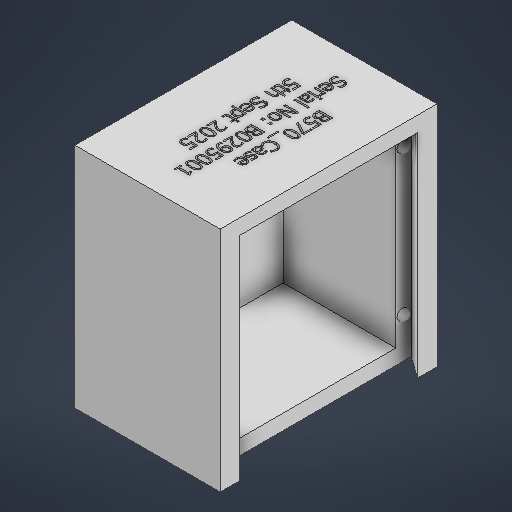
# Autodesk Inventor part: BoxCover295
Saved by Autodesk Inventor 2026.1 (Build 301233000, 233)
## iProperties
Created: 2025-09-05
Part Number: BoxCover295
Material: Generic
Document SubType Name: Modeling
Designer: usman
Density: 1 g/cm^3
Appearance: Default
Author: usman
Autodesk Inventor part; units mm, degrees
(part 1 of 2)
ref_plane "YZ Plane" through (0, 0, 0) normal (1, 0, 0) x (0, 1, 0)
ref_plane "XZ Plane" through (0, 0, 0) normal (0, 1, 0) x (-1, 0, 0)
ref_plane "XY Plane" through (0, 0, 0) normal (0, 0, 1) x (1, 0, 0)
sketch "Sketch1" plane through (0, 0, 0) normal (1, 0, 0) x (0, 1, 0)
  line L0 (-52.5, 50) -> (52.5, 50)
  line L1 (52.5, 50) -> (52.5, -50)
  line L2 (52.5, -50) -> (-52.5, -50)
  line L3 (-52.5, -50) -> (-52.5, 50)
  line L4 (-52.5, 50) -> (52.5, -50) construction
  line L5 (52.5, 50) -> (-52.5, -50) construction
  point P0 (0, 0)
  dimension "d0" = 100
  dimension "d1" = 105
  constraints: 12 end point, 2 midpoint, 2 parallel, 1 horizontal, 1 perpendicular
  measures "d0" distance of L0.end L1.end
  measures "d1" distance of L1.end L2.end
extrude "Extrusion1" add sketch "Sketch1" along normal blind 67
sketch "Sketch2" plane through (67, 0, 0) normal (1, 0, 0) x (0, 0, -1)
  line L0 (-41, -45.5) -> (41, -45.5)
  line L1 (41, -45.5) -> (41, 45.5)
  line L2 (41, 45.5) -> (-41, 45.5)
  line L3 (-41, 45.5) -> (-41, -45.5)
  line L4 (-41, -45.5) -> (41, 45.5) construction
  line L5 (41, -45.5) -> (-41, 45.5) construction
  point P0 (0, 0)
  dimension "d4" = 82
  dimension "d5" = 91
  constraints: 12 end point, 2 midpoint, 2 parallel, 1 horizontal, 1 perpendicular
  measures "d4" distance of L1.end L2.end
  measures "d5" distance of L0.end L1.end
extrude "Extrusion2" cut sketch "Sketch2" against normal blind 62
sketch "Sketch3" plane through (0, -52.5, -50) normal (0, -1, 0) x (1, 0, 0)
  point P0 (0, 50)
sketch "Sketch4" plane through (0, -52.5, -50) normal (0, -1, 0) x (1, 0, 0)
  point P0 (0, 50)
sketch "Sketch9" plane through (0, -52.5, -50) normal (0, -1, 0) x (1, 0, 0)
  line L0 (67, 9) -> (67, 91) projected
  line L1 (67, 91) -> (57, 98.0021)
  line L2 (57, 98.0021) -> (57, 1.9979)
  line L3 (57, 1.9979) -> (67, 9)
  line L4 (67, 100) -> (67, 0) projected
  point P0 (0, 50)
  dimension "d14" = 125
  dimension "d15" = 10
  dimension "d16" = 125
  constraints: 6 end point, 1 parallel
  measures "d14" angle of L4 L1
  measures "d15" distance from line of L2 L0.end
  measures "d16" angle of L3 L4
extrude "Extrusion3" cut sketch "Sketch9" against normal up to surface (98 mm away)
sketch "Sketch10" plane through (57, -52.5, 48.0021) normal (1, 0, 0) x (0, 0, -1)
  arc A0 (6.5021, 86) -> (1.5021, 86) centre (4.0021, 86) ccw
  arc A1 (94.5021, 86) -> (89.5021, 86) centre (92.0021, 86) ccw
  line L0 (7.0021, 98) -> (0, 98) projected
  line L1 (96.0042, 98) -> (89.0021, 98) projected
  line L2 (89.0021, 98) -> (89.0021, 0) projected
  line L3 (7.0021, 0) -> (7.0021, 98) projected
  line L4 (1.5021, 86) -> (6.5021, 86)
  line L5 (0, 0) -> (0, 98) projected
  line L6 (89.5021, 86) -> (94.5021, 86)
  point P0 (48.0021, 52.5)
  point P1 (3.501, 98)
  point P2 (92.5031, 98)
  dimension "d19" = 5
  dimension "d20" = 5
  dimension "d21" = 12
  dimension "d22" = 12
  dimension "d23" = 3
  dimension "d24" = 3
  constraints: 4 end point, 4 point on circle, 2 centre point, 2 midpoint, 1 horizontal, 1 perpendicular, 1 other
  measures "d19" diameter of A0
  measures "d20" diameter of A1
  measures "d21" vertical distance of point (3.501, 98) A0.centre
  measures "d22" vertical distance of point (92.503, 98) A1.centre
  measures "d23" distance from line of L2 A1.centre
  measures "d24" distance from line of L3 A0.centre
revolve "Revolution1" add sketch "Sketch10" angle 360 about axis through (57, 33.5, -41.5) along (0, 0, -1)
sketch "Sketch11" plane through (0, 52.5, 50) normal (0, 1, 0) x (1, 0, 0)
  line L0 (68.0097, 100.1192) -> (68.0097, 0.8322) construction
  line L1 (68.0097, 0.8322) -> (1.2743, 0.8322) construction
  line L2 (1.2743, 0.8322) -> (1.2743, 100.1192) construction
  line L3 (1.2743, 100.1192) -> (68.0097, 100.1192) construction
  spline S0 degree 2 poles (44.2837, 66.1356) (43.8292, 66.1356) (43.1327, 66.4814) (42.9055, 66.768) knots 0 0 0 1 2 2 2
  spline S1 degree 2 poles (42.9055, 66.768) (42.6387, 67.1138) (42.4115, 67.8992) (42.4115, 68.5217) knots 0 0 0 1 2 2 2
  line L4 (42.4115, 68.5217) -> (42.4115, 70.2704)
  line L5 (42.4115, 70.2704) -> (48.5075, 70.2704)
  line L6 (48.5075, 70.2704) -> (48.5075, 68.655)
  spline S2 degree 2 poles (48.5075, 68.655) (48.5075, 68.003) (48.4235, 67.3509) (48.2605, 67.0545) knots 0 0 0 1 2 2 2
  spline S3 degree 2 poles (48.2605, 67.0545) (48.0875, 66.7235) (47.5194, 66.4222) (47.1341, 66.4222) knots 0 0 0 1 2 2 2
  spline S4 degree 2 poles (47.1341, 66.4222) (46.7043, 66.4222) (46.0226, 66.8766) (45.83, 67.2768) knots 0 0 0 1 2 2 2
  line L7 (45.83, 67.2768) -> (45.8003, 67.2768)
  spline S5 degree 2 poles (45.8003, 67.2768) (45.6521, 66.7334) (44.8666, 66.1356) (44.2837, 66.1356) knots 0 0 0 1 2 2 2
  spline S6 degree 2 poles (44.2491, 66.9804) (44.5949, 66.9804) (45.0395, 67.178) (45.1976, 67.4744) knots 0 0 0 1 2 2 2
  spline S7 degree 2 poles (45.1976, 67.4744) (45.2964, 67.667) (45.3557, 68.1215) (45.3557, 68.5414) knots 0 0 0 1 2 2 2
  line L8 (45.3557, 68.5414) -> (45.3557, 69.4603)
  line L9 (45.3557, 69.4603) -> (43.1031, 69.4603)
  line L10 (43.1031, 69.4603) -> (43.1031, 68.8032)
  spline S8 degree 2 poles (43.1031, 68.8032) (43.1031, 68.2697) (43.2019, 67.6572) (43.3599, 67.42) knots 0 0 0 1 2 2 2
  spline S9 degree 2 poles (43.3599, 67.42) (43.523, 67.1928) (43.928, 66.9804) (44.2491, 66.9804) knots 0 0 0 1 2 2 2
  spline S10 degree 2 poles (47.0205, 67.2669) (47.2379, 67.2669) (47.5639, 67.4151) (47.6578, 67.5781) knots 0 0 0 1 2 2 2
  spline S11 degree 2 poles (47.6578, 67.5781) (47.7664, 67.7757) (47.8158, 68.2549) (47.8158, 68.6847) knots 0 0 0 1 2 2 2
  line L11 (47.8158, 68.6847) -> (47.8158, 69.4603)
  line L12 (47.8158, 69.4603) -> (46.0325, 69.4603)
  line L13 (46.0325, 69.4603) -> (46.0325, 68.5414)
  spline S12 degree 2 poles (46.0325, 68.5414) (46.0325, 68.161) (46.1115, 67.8004) (46.235, 67.6078) knots 0 0 0 1 2 2 2
  spline S13 degree 2 poles (46.235, 67.6078) (46.3536, 67.42) (46.734, 67.2669) (47.0205, 67.2669) knots 0 0 0 1 2 2 2
  spline S14 degree 2 poles (44.3479, 61.8082) (43.9083, 61.8082) (43.1574, 62.0897) (42.8808, 62.3466) knots 0 0 0 1 2 2 2
  spline S15 degree 2 poles (42.8808, 62.3466) (42.6041, 62.6035) (42.283, 63.3692) (42.283, 63.8435) knots 0 0 0 1 2 2 2
  spline S16 degree 2 poles (42.283, 63.8435) (42.283, 64.2782) (42.4757, 65.1279) (42.6288, 65.4391) knots 0 0 0 1 2 2 2
  line L14 (42.6288, 65.4391) -> (43.4933, 65.4391)
  line L15 (43.4933, 65.4391) -> (43.4933, 65.3798)
  spline S17 degree 2 poles (43.4933, 65.3798) (43.4242, 65.2859) (43.2463, 64.9352) (43.1673, 64.7228) knots 0 0 0 1 2 2 2
  spline S18 degree 2 poles (43.1673, 64.7228) (43.0833, 64.4807) (42.9894, 64.0806) (42.9894, 63.8286) knots 0 0 0 1 2 2 2
  spline S19 degree 2 poles (42.9894, 63.8286) (42.9894, 63.5816) (43.1673, 63.1173) (43.3599, 62.9493) knots 0 0 0 1 2 2 2
  spline S20 degree 2 poles (43.3599, 62.9493) (43.5427, 62.7962) (44.0268, 62.6381) (44.3529, 62.6381) knots 0 0 0 1 2 2 2
  spline S21 degree 2 poles (44.3529, 62.6381) (44.6789, 62.6381) (45.0939, 62.8159) (45.2322, 62.9839) knots 0 0 0 1 2 2 2
  spline S22 degree 2 poles (45.2322, 62.9839) (45.3854, 63.1568) (45.5138, 63.6706) (45.5138, 63.9818) knots 0 0 0 1 2 2 2
  spline S23 degree 2 poles (45.5138, 63.9818) (45.5138, 64.3177) (45.4101, 64.9846) (45.3656, 65.1871) knots 0 0 0 1 2 2 2
  line L16 (45.3656, 65.1871) -> (48.5075, 65.1871)
  line L17 (48.5075, 65.1871) -> (48.5075, 61.8427)
  line L18 (48.5075, 61.8427) -> (47.7911, 61.8427)
  line L19 (47.7911, 61.8427) -> (47.7911, 64.4017)
  line L20 (47.7911, 64.4017) -> (46.1659, 64.4017)
  spline S24 degree 2 poles (46.1659, 64.4017) (46.1856, 64.2535) (46.2005, 63.967) (46.2005, 63.8484) knots 0 0 0 1 2 2 2
  spline S25 degree 2 poles (46.2005, 63.8484) (46.2005, 63.3791) (46.0473, 62.732) (45.8201, 62.4355) knots 0 0 0 1 2 2 2
  spline S26 degree 2 poles (45.8201, 62.4355) (45.5928, 62.1342) (44.9012, 61.8082) (44.3479, 61.8082) knots 0 0 0 1 2 2 2
  line L21 (47.5935, 57.1003) -> (42.4115, 59.7383)
  line L22 (42.4115, 59.7383) -> (42.4115, 60.6077)
  line L23 (42.4115, 60.6077) -> (47.7911, 57.8216)
  line L24 (47.7911, 57.8216) -> (47.7911, 60.9684)
  line L25 (47.7911, 60.9684) -> (48.5075, 60.9684)
  line L26 (48.5075, 60.9684) -> (48.5075, 57.1003)
  line L27 (48.5075, 57.1003) -> (47.5935, 57.1003)
  spline S27 degree 2 poles (45.4595, 52.5604) (43.8194, 52.5604) (42.283, 53.5138) (42.283, 54.5068) knots 0 0 0 1 2 2 2
  spline S28 degree 2 poles (42.283, 54.5068) (42.283, 55.5146) (43.849, 56.4581) (45.4545, 56.4581) knots 0 0 0 1 2 2 2
  spline S29 degree 2 poles (45.4545, 56.4581) (47.1045, 56.4581) (48.631, 55.5047) (48.631, 54.5068) knots 0 0 0 1 2 2 2
  spline S30 degree 2 poles (48.631, 54.5068) (48.631, 53.504) (47.0501, 52.5604) (45.4595, 52.5604) knots 0 0 0 1 2 2 2
  spline S31 degree 2 poles (43.602, 53.6077) (43.9033, 53.4891) (44.8321, 53.3903) (45.4595, 53.3903) knots 0 0 0 1 2 2 2
  spline S32 degree 2 poles (45.4595, 53.3903) (46.0868, 53.3903) (47.0106, 53.4891) (47.3218, 53.6127) knots 0 0 0 1 2 2 2
  spline S33 degree 2 poles (47.3218, 53.6127) (47.6331, 53.7362) (47.9542, 54.1659) (47.9542, 54.5068) knots 0 0 0 1 2 2 2
  spline S34 degree 2 poles (47.9542, 54.5068) (47.9542, 54.8477) (47.6331, 55.2873) (47.312, 55.4158) knots 0 0 0 1 2 2 2
  spline S35 degree 2 poles (47.312, 55.4158) (47.0007, 55.5393) (46.0523, 55.6282) (45.4545, 55.6282) knots 0 0 0 1 2 2 2
  spline S36 degree 2 poles (45.4545, 55.6282) (44.8123, 55.6282) (43.9527, 55.5491) (43.6168, 55.4207) knots 0 0 0 1 2 2 2
  spline S37 degree 2 poles (43.6168, 55.4207) (43.3007, 55.3021) (42.9598, 54.8625) (42.9598, 54.5068) knots 0 0 0 1 2 2 2
  spline S38 degree 2 poles (42.9598, 54.5068) (42.9598, 54.1709) (43.2809, 53.7312) (43.602, 53.6077) knots 0 0 0 1 2 2 2
  line L28 (41.1863, 47.5858) -> (41.1863, 52.2887)
  line L29 (41.1863, 52.2887) -> (41.7149, 52.2887)
  line L30 (41.7149, 52.2887) -> (41.7149, 47.5858)
  line L31 (41.7149, 47.5858) -> (41.1863, 47.5858)
  spline S39 degree 2 poles (42.3028, 44.6514) (42.3028, 45.2442) (42.7029, 46.2471) (43.1031, 46.6126) knots 0 0 0 1 2 2 2
  spline S40 degree 2 poles (43.1031, 46.6126) (43.4983, 46.9782) (44.6839, 47.3783) (45.4545, 47.3783) knots 0 0 0 1 2 2 2
  spline S41 degree 2 poles (45.4545, 47.3783) (46.2202, 47.3783) (47.3564, 46.9881) (47.7763, 46.6176) knots 0 0 0 1 2 2 2
  spline S42 degree 2 poles (47.7763, 46.6176) (48.1864, 46.252) (48.6161, 45.2541) (48.6161, 44.6366) knots 0 0 0 1 2 2 2
  spline S43 degree 2 poles (48.6161, 44.6366) (48.6161, 44.3303) (48.5272, 43.7919) (48.4581, 43.5646) knots 0 0 0 1 2 2 2
  spline S44 degree 2 poles (48.4581, 43.5646) (48.3938, 43.367) (48.2111, 42.957) (48.1024, 42.7545) knots 0 0 0 1 2 2 2
  line L32 (48.1024, 42.7545) -> (47.1242, 42.7545)
  line L33 (47.1242, 42.7545) -> (47.1242, 42.8187)
  spline S45 degree 2 poles (47.1242, 42.8187) (47.223, 42.9274) (47.4997, 43.2633) (47.6331, 43.5053) knots 0 0 0 1 2 2 2
  spline S46 degree 2 poles (47.6331, 43.5053) (47.7615, 43.7375) (47.9245, 44.2859) (47.9245, 44.6416) knots 0 0 0 1 2 2 2
  spline S47 degree 2 poles (47.9245, 44.6416) (47.9245, 45.0318) (47.6034, 45.7284) (47.2971, 45.9902) knots 0 0 0 1 2 2 2
  spline S48 degree 2 poles (47.2971, 45.9902) (46.9859, 46.2471) (46.0424, 46.5336) (45.4545, 46.5336) knots 0 0 0 1 2 2 2
  spline S49 degree 2 poles (45.4545, 46.5336) (44.8271, 46.5336) (43.9231, 46.2322) (43.6119, 45.9704) knots 0 0 0 1 2 2 2
  spline S50 degree 2 poles (43.6119, 45.9704) (43.3105, 45.7135) (43.0043, 45.0269) (43.0043, 44.6416) knots 0 0 0 1 2 2 2
  spline S51 degree 2 poles (43.0043, 44.6416) (43.0043, 44.2908) (43.1772, 43.6931) (43.3056, 43.4609) knots 0 0 0 1 2 2 2
  spline S52 degree 2 poles (43.3056, 43.4609) (43.434, 43.2386) (43.7008, 42.9076) (43.7947, 42.8137) knots 0 0 0 1 2 2 2
  line L34 (43.7947, 42.8137) -> (43.7947, 42.7545)
  line L35 (43.7947, 42.7545) -> (42.8264, 42.7545)
  spline S53 degree 2 poles (42.8264, 42.7545) (42.7326, 42.957) (42.5597, 43.3127) (42.4806, 43.5646) knots 0 0 0 1 2 2 2
  spline S54 degree 2 poles (42.4806, 43.5646) (42.3917, 43.8314) (42.3028, 44.2859) (42.3028, 44.6514) knots 0 0 0 1 2 2 2
  spline S55 degree 2 poles (42.8956, 39.5089) (42.8264, 39.6027) (42.5794, 39.9189) (42.5053, 40.0671) knots 0 0 0 1 2 2 2
  spline S56 degree 2 poles (42.5053, 40.0671) (42.3966, 40.2696) (42.283, 40.65) (42.283, 40.9958) knots 0 0 0 1 2 2 2
  spline S57 degree 2 poles (42.283, 40.9958) (42.283, 41.2774) (42.4954, 41.7862) (42.6881, 41.9789) knots 0 0 0 1 2 2 2
  spline S58 degree 2 poles (42.6881, 41.9789) (42.8758, 42.1617) (43.4291, 42.384) (43.7354, 42.384) knots 0 0 0 1 2 2 2
  spline S59 degree 2 poles (43.7354, 42.384) (44.2096, 42.384) (44.8815, 41.9838) (45.0741, 41.5491) knots 0 0 0 1 2 2 2
  spline S60 degree 2 poles (45.0741, 41.5491) (45.252, 41.1638) (45.3854, 40.1165) (45.4199, 39.5089) knots 0 0 0 1 2 2 2
  line L36 (45.4199, 39.5089) -> (45.5681, 39.5089)
  spline S61 degree 2 poles (45.5681, 39.5089) (45.8349, 39.5089) (46.1659, 39.6719) (46.2597, 39.8201) knots 0 0 0 1 2 2 2
  spline S62 degree 2 poles (46.2597, 39.8201) (46.3536, 39.9683) (46.4129, 40.3931) (46.4129, 40.6204) knots 0 0 0 1 2 2 2
  spline S63 degree 2 poles (46.4129, 40.6204) (46.4129, 40.8871) (46.2548, 41.6084) (46.1017, 41.969) knots 0 0 0 1 2 2 2
  line L37 (46.1017, 41.969) -> (46.1017, 42.0135)
  line L38 (46.1017, 42.0135) -> (46.8871, 42.0135)
  spline S64 degree 2 poles (46.8871, 42.0135) (46.9464, 41.801) (47.0946, 41.0057) (47.0946, 40.6154) knots 0 0 0 1 2 2 2
  spline S65 degree 2 poles (47.0946, 40.6154) (47.0946, 40.1412) (46.9464, 39.494) (46.7537, 39.2372) knots 0 0 0 1 2 2 2
  spline S66 degree 2 poles (46.7537, 39.2372) (46.566, 38.9852) (45.9683, 38.7382) (45.5385, 38.7382) knots 0 0 0 1 2 2 2
  line L39 (45.5385, 38.7382) -> (42.4115, 38.7382)
  line L40 (42.4115, 38.7382) -> (42.4115, 39.5089)
  line L41 (42.4115, 39.5089) -> (42.8956, 39.5089)
  line L42 (43.5378, 39.5089) -> (44.8074, 39.5089)
  spline S67 degree 2 poles (44.8074, 39.5089) (44.7827, 39.7855) (44.6987, 40.6204) (44.6196, 40.8822) knots 0 0 0 1 2 2 2
  spline S68 degree 2 poles (44.6196, 40.8822) (44.5258, 41.1885) (44.1355, 41.5886) (43.7897, 41.5886) knots 0 0 0 1 2 2 2
  spline S69 degree 2 poles (43.7897, 41.5886) (43.3945, 41.5886) (42.9944, 41.144) (42.9944, 40.7192) knots 0 0 0 1 2 2 2
  spline S70 degree 2 poles (42.9944, 40.7192) (42.9944, 40.3585) (43.3056, 39.7657) (43.5378, 39.5089) knots 0 0 0 1 2 2 2
  spline S71 degree 2 poles (42.3028, 36.4213) (42.3028, 36.8808) (42.5498, 37.6761) (42.6881, 37.9379) knots 0 0 0 1 2 2 2
  line L43 (42.6881, 37.9379) -> (43.5526, 37.9379)
  line L44 (43.5526, 37.9379) -> (43.5526, 37.8984)
  spline S72 degree 2 poles (43.5526, 37.8984) (43.4736, 37.7996) (43.2858, 37.5328) (43.1821, 37.3105) knots 0 0 0 1 2 2 2
  spline S73 degree 2 poles (43.1821, 37.3105) (43.0882, 37.1179) (42.9499, 36.6436) (42.9499, 36.3917) knots 0 0 0 1 2 2 2
  spline S74 degree 2 poles (42.9499, 36.3917) (42.9499, 36.2089) (43.0339, 35.789) (43.1031, 35.6902) knots 0 0 0 1 2 2 2
  spline S75 degree 2 poles (43.1031, 35.6902) (43.1969, 35.547) (43.4093, 35.4185) (43.6267, 35.4185) knots 0 0 0 1 2 2 2
  spline S76 degree 2 poles (43.6267, 35.4185) (43.8984, 35.4185) (44.18, 35.7149) (44.2738, 36.0953) knots 0 0 0 1 2 2 2
  spline S77 degree 2 poles (44.2738, 36.0953) (44.3084, 36.2435) (44.4072, 36.7177) (44.4616, 36.9203) knots 0 0 0 1 2 2 2
  spline S78 degree 2 poles (44.4616, 36.9203) (44.6147, 37.4439) (45.247, 37.9182) (45.6966, 37.9182) knots 0 0 0 1 2 2 2
  spline S79 degree 2 poles (45.6966, 37.9182) (46.319, 37.9182) (47.0946, 36.9845) (47.0946, 36.2139) knots 0 0 0 1 2 2 2
  spline S80 degree 2 poles (47.0946, 36.2139) (47.0946, 35.8335) (46.9069, 35.0628) (46.7636, 34.801) knots 0 0 0 1 2 2 2
  line L45 (46.7636, 34.801) -> (45.9386, 34.801)
  line L46 (45.9386, 34.801) -> (45.9386, 34.8405)
  spline S81 degree 2 poles (45.9386, 34.8405) (46.1758, 35.1369) (46.4475, 35.8582) (46.4475, 36.2287) knots 0 0 0 1 2 2 2
  spline S82 degree 2 poles (46.4475, 36.2287) (46.4475, 36.6091) (46.1264, 37.1327) (45.8053, 37.1327) knots 0 0 0 1 2 2 2
  spline S83 degree 2 poles (45.8053, 37.1327) (45.5138, 37.1327) (45.2322, 36.8215) (45.1433, 36.4757) knots 0 0 0 1 2 2 2
  spline S84 degree 2 poles (45.1433, 36.4757) (45.0988, 36.3077) (45.0099, 35.8829) (44.9556, 35.6507) knots 0 0 0 1 2 2 2
  spline S85 degree 2 poles (44.9556, 35.6507) (44.8271, 35.1468) (44.2393, 34.633) (43.7304, 34.633) knots 0 0 0 1 2 2 2
  spline S86 degree 2 poles (43.7304, 34.633) (43.434, 34.633) (42.9104, 34.8652) (42.7177, 35.0925) knots 0 0 0 1 2 2 2
  spline S87 degree 2 poles (42.7177, 35.0925) (42.5152, 35.3345) (42.3028, 35.952) (42.3028, 36.4213) knots 0 0 0 1 2 2 2
  spline S88 degree 2 poles (42.3077, 31.9308) (42.3077, 33.0275) (43.5378, 34.2329) (44.674, 34.2329) knots 0 0 0 1 2 2 2
  spline S89 degree 2 poles (44.674, 34.2329) (45.7904, 34.2329) (47.1144, 33.0621) (47.1144, 32.1186) knots 0 0 0 1 2 2 2
  spline S90 degree 2 poles (47.1144, 32.1186) (47.1144, 31.6937) (46.8674, 31.0367) (46.6055, 30.7946) knots 0 0 0 1 2 2 2
  spline S91 degree 2 poles (46.6055, 30.7946) (46.3437, 30.5476) (45.5879, 30.2858) (45.0395, 30.2858) knots 0 0 0 1 2 2 2
  line L47 (45.0395, 30.2858) -> (44.6196, 30.2858)
  line L48 (44.6196, 30.2858) -> (44.6196, 33.4524)
  spline S92 degree 2 poles (44.6196, 33.4524) (43.8243, 33.4524) (42.9796, 32.6521) (42.9796, 31.9407) knots 0 0 0 1 2 2 2
  spline S93 degree 2 poles (42.9796, 31.9407) (42.9796, 31.6888) (43.0932, 31.1997) (43.1821, 31.0021) knots 0 0 0 1 2 2 2
  spline S94 degree 2 poles (43.1821, 31.0021) (43.2809, 30.7946) (43.4538, 30.5081) (43.5328, 30.4143) knots 0 0 0 1 2 2 2
  line L49 (43.5328, 30.4143) -> (43.5328, 30.3698)
  line L50 (43.5328, 30.3698) -> (42.693, 30.3698)
  spline S95 degree 2 poles (42.693, 30.3698) (42.6387, 30.5032) (42.4806, 30.9083) (42.4362, 31.0663) knots 0 0 0 1 2 2 2
  spline S96 degree 2 poles (42.4362, 31.0663) (42.3719, 31.2886) (42.3077, 31.6542) (42.3077, 31.9308) knots 0 0 0 1 2 2 2
  spline S97 degree 2 poles (45.2075, 31.0367) (45.5187, 31.0466) (45.9732, 31.175) (46.1264, 31.2985) knots 0 0 0 1 2 2 2
  spline S98 degree 2 poles (46.1264, 31.2985) (46.2993, 31.4319) (46.482, 31.8518) (46.482, 32.163) knots 0 0 0 1 2 2 2
  spline S99 degree 2 poles (46.482, 32.163) (46.482, 32.4693) (46.2993, 32.8991) (46.1214, 33.0769) knots 0 0 0 1 2 2 2
  spline S100 degree 2 poles (46.1214, 33.0769) (45.9386, 33.2498) (45.499, 33.4277) (45.2075, 33.4524) knots 0 0 0 1 2 2 2
  line L51 (45.2075, 33.4524) -> (45.2075, 31.0367)
  spline S101 degree 2 poles (32.2659, 85.9822) (32.2659, 86.6442) (32.5425, 87.5729) (32.7401, 87.9829) knots 0 0 0 1 2 2 2
  line L52 (32.7401, 87.9829) -> (33.7578, 87.9829)
  line L53 (33.7578, 87.9829) -> (33.7578, 87.9236)
  spline S102 degree 2 poles (33.7578, 87.9236) (33.3823, 87.5235) (32.9674, 86.5108) (32.9674, 86.0415) knots 0 0 0 1 2 2 2
  spline S103 degree 2 poles (32.9674, 86.0415) (32.9674, 85.3696) (33.5256, 84.683) (33.985, 84.683) knots 0 0 0 1 2 2 2
  spline S104 degree 2 poles (33.985, 84.683) (34.3506, 84.683) (34.805, 85.0436) (34.9187, 85.4339) knots 0 0 0 1 2 2 2
  spline S105 degree 2 poles (34.9187, 85.4339) (34.9977, 85.7155) (35.1064, 86.1848) (35.1953, 86.5355) knots 0 0 0 1 2 2 2
  spline S106 degree 2 poles (35.1953, 86.5355) (35.2793, 86.8517) (35.5312, 87.3506) (35.7338, 87.5433) knots 0 0 0 1 2 2 2
  spline S107 degree 2 poles (35.7338, 87.5433) (35.9363, 87.731) (36.4797, 87.9385) (36.8354, 87.9385) knots 0 0 0 1 2 2 2
  spline S108 degree 2 poles (36.8354, 87.9385) (37.5764, 87.9385) (38.5792, 86.7825) (38.5792, 85.8884) knots 0 0 0 1 2 2 2
  spline S109 degree 2 poles (38.5792, 85.8884) (38.5792, 85.3746) (38.3767, 84.4656) (38.184, 84.0754) knots 0 0 0 1 2 2 2
  line L54 (38.184, 84.0754) -> (37.2158, 84.0754)
  line L55 (37.2158, 84.0754) -> (37.2158, 84.1346)
  spline S110 degree 2 poles (37.2158, 84.1346) (37.4825, 84.4261) (37.8777, 85.3351) (37.8777, 85.834) knots 0 0 0 1 2 2 2
  spline S111 degree 2 poles (37.8777, 85.834) (37.8777, 86.3972) (37.3492, 87.0937) (36.9194, 87.0937) knots 0 0 0 1 2 2 2
  spline S112 degree 2 poles (36.9194, 87.0937) (36.5341, 87.0937) (36.0746, 86.6837) (35.9709, 86.2984) knots 0 0 0 1 2 2 2
  spline S113 degree 2 poles (35.9709, 86.2984) (35.9017, 86.0415) (35.7239, 85.2955) (35.6498, 85.0485) knots 0 0 0 1 2 2 2
  spline S114 degree 2 poles (35.6498, 85.0485) (35.4571, 84.4212) (34.6815, 83.8382) (34.1134, 83.8382) knots 0 0 0 1 2 2 2
  spline S115 degree 2 poles (34.1134, 83.8382) (33.7528, 83.8382) (33.0612, 84.1297) (32.8192, 84.3915) knots 0 0 0 1 2 2 2
  spline S116 degree 2 poles (32.8192, 84.3915) (32.5524, 84.683) (32.2659, 85.424) (32.2659, 85.9822) knots 0 0 0 1 2 2 2
  spline S117 degree 2 poles (32.2708, 81.0866) (32.2708, 82.1833) (33.5009, 83.3887) (34.6371, 83.3887) knots 0 0 0 1 2 2 2
  spline S118 degree 2 poles (34.6371, 83.3887) (35.7535, 83.3887) (37.0775, 82.2179) (37.0775, 81.2744) knots 0 0 0 1 2 2 2
  spline S119 degree 2 poles (37.0775, 81.2744) (37.0775, 80.8495) (36.8305, 80.1925) (36.5686, 79.9504) knots 0 0 0 1 2 2 2
  spline S120 degree 2 poles (36.5686, 79.9504) (36.3068, 79.7034) (35.551, 79.4416) (35.0026, 79.4416) knots 0 0 0 1 2 2 2
  line L56 (35.0026, 79.4416) -> (34.5827, 79.4416)
  line L57 (34.5827, 79.4416) -> (34.5827, 82.6082)
  spline S121 degree 2 poles (34.5827, 82.6082) (33.7874, 82.6082) (32.9427, 81.8079) (32.9427, 81.0965) knots 0 0 0 1 2 2 2
  spline S122 degree 2 poles (32.9427, 81.0965) (32.9427, 80.8446) (33.0563, 80.3555) (33.1452, 80.1579) knots 0 0 0 1 2 2 2
  spline S123 degree 2 poles (33.1452, 80.1579) (33.244, 79.9504) (33.4169, 79.6639) (33.4959, 79.5701) knots 0 0 0 1 2 2 2
  line L58 (33.4959, 79.5701) -> (33.4959, 79.5256)
  line L59 (33.4959, 79.5256) -> (32.6561, 79.5256)
  spline S124 degree 2 poles (32.6561, 79.5256) (32.6018, 79.659) (32.4437, 80.0641) (32.3992, 80.2221) knots 0 0 0 1 2 2 2
  spline S125 degree 2 poles (32.3992, 80.2221) (32.335, 80.4444) (32.2708, 80.81) (32.2708, 81.0866) knots 0 0 0 1 2 2 2
  spline S126 degree 2 poles (35.1706, 80.1925) (35.4818, 80.2024) (35.9363, 80.3308) (36.0895, 80.4543) knots 0 0 0 1 2 2 2
  spline S127 degree 2 poles (36.0895, 80.4543) (36.2624, 80.5877) (36.4451, 81.0076) (36.4451, 81.3188) knots 0 0 0 1 2 2 2
  spline S128 degree 2 poles (36.4451, 81.3188) (36.4451, 81.6251) (36.2624, 82.0549) (36.0845, 82.2327) knots 0 0 0 1 2 2 2
  spline S129 degree 2 poles (36.0845, 82.2327) (35.9017, 82.4056) (35.4621, 82.5835) (35.1706, 82.6082) knots 0 0 0 1 2 2 2
  line L60 (35.1706, 82.6082) -> (35.1706, 80.1925)
  line L61 (36.124, 76.2355) -> (36.124, 76.275)
  spline S130 degree 2 poles (36.124, 76.275) (36.1487, 76.364) (36.1586, 76.5566) (36.1586, 76.69) knots 0 0 0 1 2 2 2
  spline S131 degree 2 poles (36.1586, 76.69) (36.1586, 77.0012) (35.8869, 77.6138) (35.6202, 77.8904) knots 0 0 0 1 2 2 2
  line L62 (35.6202, 77.8904) -> (32.3745, 77.8904)
  line L63 (32.3745, 77.8904) -> (32.3745, 78.6611)
  line L64 (32.3745, 78.6611) -> (36.949, 78.6611)
  line L65 (36.949, 78.6611) -> (36.949, 77.8904)
  line L66 (36.949, 77.8904) -> (36.2673, 77.8904)
  spline S132 degree 2 poles (36.2673, 77.8904) (36.6427, 77.4705) (36.949, 76.8432) (36.949, 76.5468) knots 0 0 0 1 2 2 2
  spline S133 degree 2 poles (36.949, 76.5468) (36.949, 76.4282) (36.9391, 76.3096) (36.9243, 76.2355) knots 0 0 0 1 2 2 2
  line L67 (36.9243, 76.2355) -> (36.124, 76.2355)
  line L68 (32.3745, 74.8523) -> (32.3745, 75.623)
  line L69 (32.3745, 75.623) -> (36.949, 75.623)
  line L70 (36.949, 75.623) -> (36.949, 74.8523)
  line L71 (36.949, 74.8523) -> (32.3745, 74.8523)
  line L72 (37.7098, 74.798) -> (37.7098, 75.6724)
  line L73 (37.7098, 75.6724) -> (38.5101, 75.6724)
  line L74 (38.5101, 75.6724) -> (38.5101, 74.798)
  line L75 (38.5101, 74.798) -> (37.7098, 74.798)
  spline S134 degree 2 poles (32.8587, 71.172) (32.7895, 71.2659) (32.5425, 71.582) (32.4684, 71.7302) knots 0 0 0 1 2 2 2
  spline S135 degree 2 poles (32.4684, 71.7302) (32.3597, 71.9328) (32.2461, 72.3131) (32.2461, 72.6589) knots 0 0 0 1 2 2 2
  spline S136 degree 2 poles (32.2461, 72.6589) (32.2461, 72.9405) (32.4585, 73.4493) (32.6512, 73.642) knots 0 0 0 1 2 2 2
  spline S137 degree 2 poles (32.6512, 73.642) (32.8389, 73.8248) (33.3922, 74.0471) (33.6985, 74.0471) knots 0 0 0 1 2 2 2
  spline S138 degree 2 poles (33.6985, 74.0471) (34.1727, 74.0471) (34.8446, 73.647) (35.0372, 73.2122) knots 0 0 0 1 2 2 2
  spline S139 degree 2 poles (35.0372, 73.2122) (35.2151, 72.8269) (35.3484, 71.7796) (35.383, 71.172) knots 0 0 0 1 2 2 2
  line L76 (35.383, 71.172) -> (35.5312, 71.172)
  spline S140 degree 2 poles (35.5312, 71.172) (35.798, 71.172) (36.129, 71.335) (36.2228, 71.4832) knots 0 0 0 1 2 2 2
  spline S141 degree 2 poles (36.2228, 71.4832) (36.3167, 71.6314) (36.376, 72.0563) (36.376, 72.2835) knots 0 0 0 1 2 2 2
  spline S142 degree 2 poles (36.376, 72.2835) (36.376, 72.5503) (36.2179, 73.2715) (36.0648, 73.6321) knots 0 0 0 1 2 2 2
  line L77 (36.0648, 73.6321) -> (36.0648, 73.6766)
  line L78 (36.0648, 73.6766) -> (36.8502, 73.6766)
  spline S143 degree 2 poles (36.8502, 73.6766) (36.9095, 73.4642) (37.0577, 72.6688) (37.0577, 72.2786) knots 0 0 0 1 2 2 2
  spline S144 degree 2 poles (37.0577, 72.2786) (37.0577, 71.8043) (36.9095, 71.1572) (36.7168, 70.9003) knots 0 0 0 1 2 2 2
  spline S145 degree 2 poles (36.7168, 70.9003) (36.5291, 70.6484) (35.9314, 70.4013) (35.5016, 70.4013) knots 0 0 0 1 2 2 2
  line L79 (35.5016, 70.4013) -> (32.3745, 70.4013)
  line L80 (32.3745, 70.4013) -> (32.3745, 71.172)
  line L81 (32.3745, 71.172) -> (32.8587, 71.172)
  line L82 (33.5009, 71.172) -> (34.7705, 71.172)
  spline S146 degree 2 poles (34.7705, 71.172) (34.7458, 71.4486) (34.6618, 72.2835) (34.5827, 72.5453) knots 0 0 0 1 2 2 2
  spline S147 degree 2 poles (34.5827, 72.5453) (34.4889, 72.8516) (34.0986, 73.2517) (33.7528, 73.2517) knots 0 0 0 1 2 2 2
  spline S148 degree 2 poles (33.7528, 73.2517) (33.3576, 73.2517) (32.9575, 72.8071) (32.9575, 72.3823) knots 0 0 0 1 2 2 2
  spline S149 degree 2 poles (32.9575, 72.3823) (32.9575, 72.0217) (33.2687, 71.4289) (33.5009, 71.172) knots 0 0 0 1 2 2 2
  line L83 (32.3745, 68.534) -> (32.3745, 69.3047)
  line L84 (32.3745, 69.3047) -> (38.7423, 69.3047)
  line L85 (38.7423, 69.3047) -> (38.7423, 68.534)
  line L86 (38.7423, 68.534) -> (32.3745, 68.534)
  line L87 (32.3745, 60.3632) -> (32.3745, 61.2722)
  line L88 (32.3745, 61.2722) -> (37.6307, 63.9694)
  line L89 (37.6307, 63.9694) -> (32.3745, 63.9694)
  line L90 (32.3745, 63.9694) -> (32.3745, 64.7253)
  line L91 (32.3745, 64.7253) -> (38.4705, 64.7253)
  line L92 (38.4705, 64.7253) -> (38.4705, 63.5742)
  line L93 (38.4705, 63.5742) -> (33.6441, 61.119)
  line L94 (33.6441, 61.119) -> (38.4705, 61.119)
  line L95 (38.4705, 61.119) -> (38.4705, 60.3632)
  line L96 (38.4705, 60.3632) -> (32.3745, 60.3632)
  spline S150 degree 2 poles (34.6618, 55.4281) (33.5058, 55.4281) (32.2461, 56.5396) (32.2461, 57.4683) knots 0 0 0 1 2 2 2
  spline S151 degree 2 poles (32.2461, 57.4683) (32.2461, 58.4218) (33.5453, 59.5135) (34.6618, 59.5135) knots 0 0 0 1 2 2 2
  spline S152 degree 2 poles (34.6618, 59.5135) (35.8079, 59.5135) (37.0775, 58.3872) (37.0775, 57.4683) knots 0 0 0 1 2 2 2
  spline S153 degree 2 poles (37.0775, 57.4683) (37.0775, 56.5396) (35.8128, 55.4281) (34.6618, 55.4281) knots 0 0 0 1 2 2 2
  spline S154 degree 2 poles (34.6618, 56.2235) (35.551, 56.2235) (36.4155, 56.8706) (36.4155, 57.4683) knots 0 0 0 1 2 2 2
  spline S155 degree 2 poles (36.4155, 57.4683) (36.4155, 58.0661) (35.551, 58.7182) (34.6618, 58.7182) knots 0 0 0 1 2 2 2
  spline S156 degree 2 poles (34.6618, 58.7182) (33.7973, 58.7182) (32.9081, 58.0661) (32.9081, 57.4683) knots 0 0 0 1 2 2 2
  spline S157 degree 2 poles (32.9081, 57.4683) (32.9081, 56.8755) (33.7825, 56.2235) (34.6618, 56.2235) knots 0 0 0 1 2 2 2
  line L97 (32.3745, 53.2249) -> (32.3745, 54.203)
  line L98 (32.3745, 54.203) -> (33.5404, 54.203)
  line L99 (33.5404, 54.203) -> (33.5404, 53.2249)
  line L100 (33.5404, 53.2249) -> (32.3745, 53.2249)
  line L101 (35.7832, 53.2249) -> (35.7832, 54.203)
  line L102 (35.7832, 54.203) -> (36.949, 54.203)
  line L103 (36.949, 54.203) -> (36.949, 53.2249)
  line L104 (36.949, 53.2249) -> (35.7832, 53.2249)
  spline S158 degree 2 poles (34.2468, 44.8614) (33.7923, 44.8614) (33.0958, 45.2072) (32.8686, 45.4937) knots 0 0 0 1 2 2 2
  spline S159 degree 2 poles (32.8686, 45.4937) (32.6018, 45.8395) (32.3745, 46.625) (32.3745, 47.2474) knots 0 0 0 1 2 2 2
  line L105 (32.3745, 47.2474) -> (32.3745, 48.9962)
  line L106 (32.3745, 48.9962) -> (38.4705, 48.9962)
  line L107 (38.4705, 48.9962) -> (38.4705, 47.3808)
  spline S160 degree 2 poles (38.4705, 47.3808) (38.4705, 46.7287) (38.3866, 46.0766) (38.2235, 45.7802) knots 0 0 0 1 2 2 2
  spline S161 degree 2 poles (38.2235, 45.7802) (38.0506, 45.4492) (37.4825, 45.1479) (37.0972, 45.1479) knots 0 0 0 1 2 2 2
  spline S162 degree 2 poles (37.0972, 45.1479) (36.6674, 45.1479) (35.9857, 45.6024) (35.7931, 46.0025) knots 0 0 0 1 2 2 2
  line L108 (35.7931, 46.0025) -> (35.7634, 46.0025)
  spline S163 degree 2 poles (35.7634, 46.0025) (35.6152, 45.4591) (34.8297, 44.8614) (34.2468, 44.8614) knots 0 0 0 1 2 2 2
  spline S164 degree 2 poles (34.2122, 45.7061) (34.558, 45.7061) (35.0026, 45.9037) (35.1607, 46.2001) knots 0 0 0 1 2 2 2
  spline S165 degree 2 poles (35.1607, 46.2001) (35.2595, 46.3928) (35.3188, 46.8473) (35.3188, 47.2672) knots 0 0 0 1 2 2 2
  line L109 (35.3188, 47.2672) -> (35.3188, 48.186)
  line L110 (35.3188, 48.186) -> (33.0662, 48.186)
  line L111 (33.0662, 48.186) -> (33.0662, 47.529)
  spline S166 degree 2 poles (33.0662, 47.529) (33.0662, 46.9955) (33.165, 46.3829) (33.323, 46.1458) knots 0 0 0 1 2 2 2
  spline S167 degree 2 poles (33.323, 46.1458) (33.4861, 45.9185) (33.8911, 45.7061) (34.2122, 45.7061) knots 0 0 0 1 2 2 2
  spline S168 degree 2 poles (36.9836, 45.9926) (37.201, 45.9926) (37.527, 46.1409) (37.6209, 46.3039) knots 0 0 0 1 2 2 2
  spline S169 degree 2 poles (37.6209, 46.3039) (37.7295, 46.5015) (37.7789, 46.9807) (37.7789, 47.4104) knots 0 0 0 1 2 2 2
  line L112 (37.7789, 47.4104) -> (37.7789, 48.186)
  line L113 (37.7789, 48.186) -> (35.9956, 48.186)
  line L114 (35.9956, 48.186) -> (35.9956, 47.2672)
  spline S170 degree 2 poles (35.9956, 47.2672) (35.9956, 46.8868) (36.0746, 46.5262) (36.1981, 46.3335) knots 0 0 0 1 2 2 2
  spline S171 degree 2 poles (36.1981, 46.3335) (36.3167, 46.1458) (36.6971, 45.9926) (36.9836, 45.9926) knots 0 0 0 1 2 2 2
  spline S172 degree 2 poles (35.4225, 40.4351) (33.7825, 40.4351) (32.2461, 41.3885) (32.2461, 42.3815) knots 0 0 0 1 2 2 2
  spline S173 degree 2 poles (32.2461, 42.3815) (32.2461, 43.3893) (33.8121, 44.3328) (35.4176, 44.3328) knots 0 0 0 1 2 2 2
  spline S174 degree 2 poles (35.4176, 44.3328) (37.0676, 44.3328) (38.594, 43.3794) (38.594, 42.3815) knots 0 0 0 1 2 2 2
  spline S175 degree 2 poles (38.594, 42.3815) (38.594, 41.3787) (37.0132, 40.4351) (35.4225, 40.4351) knots 0 0 0 1 2 2 2
  spline S176 degree 2 poles (33.5651, 41.4824) (33.8664, 41.3638) (34.7952, 41.265) (35.4225, 41.265) knots 0 0 0 1 2 2 2
  spline S177 degree 2 poles (35.4225, 41.265) (36.0499, 41.265) (36.9737, 41.3638) (37.2849, 41.4873) knots 0 0 0 1 2 2 2
  spline S178 degree 2 poles (37.2849, 41.4873) (37.5962, 41.6108) (37.9173, 42.0406) (37.9173, 42.3815) knots 0 0 0 1 2 2 2
  spline S179 degree 2 poles (37.9173, 42.3815) (37.9173, 42.7223) (37.5962, 43.162) (37.2751, 43.2905) knots 0 0 0 1 2 2 2
  spline S180 degree 2 poles (37.2751, 43.2905) (36.9638, 43.414) (36.0154, 43.5029) (35.4176, 43.5029) knots 0 0 0 1 2 2 2
  spline S181 degree 2 poles (35.4176, 43.5029) (34.7754, 43.5029) (33.9158, 43.4238) (33.5799, 43.2954) knots 0 0 0 1 2 2 2
  spline S182 degree 2 poles (33.5799, 43.2954) (33.2638, 43.1768) (32.9229, 42.7372) (32.9229, 42.3815) knots 0 0 0 1 2 2 2
  spline S183 degree 2 poles (32.9229, 42.3815) (32.9229, 42.0456) (33.244, 41.6059) (33.5651, 41.4824) knots 0 0 0 1 2 2 2
  line L115 (32.3745, 35.8952) -> (32.3745, 39.6546)
  line L116 (32.3745, 39.6546) -> (33.2391, 39.6546)
  spline S184 degree 2 poles (33.2391, 39.6546) (33.6194, 39.2495) (34.3259, 38.5283) (34.7062, 38.1825) knots 0 0 0 1 2 2 2
  spline S185 degree 2 poles (34.7062, 38.1825) (35.4719, 37.4859) (36.3908, 36.9771) (36.8799, 36.9771) knots 0 0 0 1 2 2 2
  spline S186 degree 2 poles (36.8799, 36.9771) (37.1367, 36.9771) (37.5221, 37.1352) (37.6456, 37.2784) knots 0 0 0 1 2 2 2
  spline S187 degree 2 poles (37.6456, 37.2784) (37.7691, 37.4217) (37.8926, 37.7971) (37.8926, 38.0244) knots 0 0 0 1 2 2 2
  spline S188 degree 2 poles (37.8926, 38.0244) (37.8926, 38.2417) (37.7839, 38.6863) (37.6999, 38.8889) knots 0 0 0 1 2 2 2
  spline S189 degree 2 poles (37.6999, 38.8889) (37.6307, 39.0618) (37.4331, 39.3829) (37.364, 39.4817) knots 0 0 0 1 2 2 2
  line L117 (37.364, 39.4817) -> (37.364, 39.5261)
  line L118 (37.364, 39.5261) -> (38.2334, 39.5261)
  spline S190 degree 2 poles (38.2334, 39.5261) (38.3569, 39.2742) (38.599, 38.3702) (38.599, 37.9651) knots 0 0 0 1 2 2 2
  spline S191 degree 2 poles (38.599, 37.9651) (38.599, 37.1105) (37.695, 36.1472) (36.9243, 36.1472) knots 0 0 0 1 2 2 2
  spline S192 degree 2 poles (36.9243, 36.1472) (36.5637, 36.1472) (35.961, 36.3151) (35.7041, 36.4633) knots 0 0 0 1 2 2 2
  spline S193 degree 2 poles (35.7041, 36.4633) (35.4374, 36.6115) (34.9137, 37.0413) (34.6618, 37.2784) knots 0 0 0 1 2 2 2
  spline S194 degree 2 poles (34.6618, 37.2784) (34.2419, 37.6638) (33.3428, 38.6073) (33.081, 38.8889) knots 0 0 0 1 2 2 2
  line L119 (33.081, 38.8889) -> (33.081, 35.8952)
  line L120 (33.081, 35.8952) -> (32.3745, 35.8952)
  spline S195 degree 2 poles (36.4896, 35.2481) (36.9589, 35.2481) (37.7394, 34.9418) (38.021, 34.675) knots 0 0 0 1 2 2 2
  spline S196 degree 2 poles (38.021, 34.675) (38.2927, 34.4231) (38.594, 33.687) (38.594, 33.3116) knots 0 0 0 1 2 2 2
  spline S197 degree 2 poles (38.594, 33.3116) (38.594, 32.8917) (38.3125, 32.21) (38.0457, 31.958) knots 0 0 0 1 2 2 2
  spline S198 degree 2 poles (38.0457, 31.958) (37.7098, 31.6419) (36.623, 31.2961) (35.7881, 31.2961) knots 0 0 0 1 2 2 2
  spline S199 degree 2 poles (35.7881, 31.2961) (35.0323, 31.2961) (33.6787, 31.6369) (33.2292, 31.9679) knots 0 0 0 1 2 2 2
  spline S200 degree 2 poles (33.2292, 31.9679) (32.7549, 32.3186) (32.256, 33.3066) (32.256, 34.0279) knots 0 0 0 1 2 2 2
  spline S201 degree 2 poles (32.256, 34.0279) (32.256, 34.1909) (32.2906, 34.5614) (32.34, 34.7195) knots 0 0 0 1 2 2 2
  line L121 (32.34, 34.7195) -> (33.1254, 34.7195)
  line L122 (33.1254, 34.7195) -> (33.1254, 34.68)
  spline S202 degree 2 poles (33.1254, 34.68) (33.0662, 34.5762) (32.9624, 34.1415) (32.9624, 33.9192) knots 0 0 0 1 2 2 2
  spline S203 degree 2 poles (32.9624, 33.9192) (32.9624, 33.1189) (34.0196, 32.205) (34.9977, 32.1408) knots 0 0 0 1 2 2 2
  spline S204 degree 2 poles (34.9977, 32.1408) (34.7754, 32.4668) (34.5729, 33.0596) (34.5729, 33.4104) knots 0 0 0 1 2 2 2
  spline S205 degree 2 poles (34.5729, 33.4104) (34.5729, 33.7463) (34.7211, 34.3045) (34.9335, 34.5861) knots 0 0 0 1 2 2 2
  spline S206 degree 2 poles (34.9335, 34.5861) (35.1854, 34.9122) (35.9511, 35.2481) (36.4896, 35.2481) knots 0 0 0 1 2 2 2
  spline S207 degree 2 poles (35.9709, 32.121) (36.5884, 32.121) (37.3689, 32.3483) (37.5813, 32.5508) knots 0 0 0 1 2 2 2
  spline S208 degree 2 poles (37.5813, 32.5508) (37.7789, 32.7287) (37.9271, 33.0992) (37.9271, 33.3165) knots 0 0 0 1 2 2 2
  spline S209 degree 2 poles (37.9271, 33.3165) (37.9271, 33.8204) (37.2059, 34.4182) (36.5242, 34.4182) knots 0 0 0 1 2 2 2
  spline S210 degree 2 poles (36.5242, 34.4182) (36.1389, 34.4182) (35.6399, 34.2206) (35.4621, 34.0032) knots 0 0 0 1 2 2 2
  spline S211 degree 2 poles (35.4621, 34.0032) (35.3336, 33.8451) (35.2496, 33.4548) (35.2496, 33.2276) knots 0 0 0 1 2 2 2
  spline S212 degree 2 poles (35.2496, 33.2276) (35.2496, 32.9658) (35.4324, 32.3631) (35.5856, 32.1359) knots 0 0 0 1 2 2 2
  spline S213 degree 2 poles (35.5856, 32.1359) (35.6449, 32.1309) (35.8474, 32.121) (35.9709, 32.121) knots 0 0 0 1 2 2 2
  spline S214 degree 2 poles (34.311, 26.8105) (33.8714, 26.8105) (33.1205, 27.0921) (32.8439, 27.349) knots 0 0 0 1 2 2 2
  spline S215 degree 2 poles (32.8439, 27.349) (32.5672, 27.6058) (32.2461, 28.3716) (32.2461, 28.8458) knots 0 0 0 1 2 2 2
  spline S216 degree 2 poles (32.2461, 28.8458) (32.2461, 29.2805) (32.4388, 30.1302) (32.5919, 30.4414) knots 0 0 0 1 2 2 2
  line L123 (32.5919, 30.4414) -> (33.4564, 30.4414)
  line L124 (33.4564, 30.4414) -> (33.4564, 30.3821)
  spline S217 degree 2 poles (33.4564, 30.3821) (33.3873, 30.2883) (33.2094, 29.9375) (33.1304, 29.7251) knots 0 0 0 1 2 2 2
  spline S218 degree 2 poles (33.1304, 29.7251) (33.0464, 29.4831) (32.9525, 29.0829) (32.9525, 28.831) knots 0 0 0 1 2 2 2
  spline S219 degree 2 poles (32.9525, 28.831) (32.9525, 28.584) (33.1304, 28.1196) (33.323, 27.9517) knots 0 0 0 1 2 2 2
  spline S220 degree 2 poles (33.323, 27.9517) (33.5058, 27.7985) (33.9899, 27.6404) (34.316, 27.6404) knots 0 0 0 1 2 2 2
  spline S221 degree 2 poles (34.316, 27.6404) (34.642, 27.6404) (35.057, 27.8183) (35.1953, 27.9862) knots 0 0 0 1 2 2 2
  spline S222 degree 2 poles (35.1953, 27.9862) (35.3484, 28.1591) (35.4769, 28.6729) (35.4769, 28.9841) knots 0 0 0 1 2 2 2
  spline S223 degree 2 poles (35.4769, 28.9841) (35.4769, 29.32) (35.3731, 29.9869) (35.3287, 30.1895) knots 0 0 0 1 2 2 2
  line L125 (35.3287, 30.1895) -> (38.4705, 30.1895)
  line L126 (38.4705, 30.1895) -> (38.4705, 26.8451)
  line L127 (38.4705, 26.8451) -> (37.7542, 26.8451)
  line L128 (37.7542, 26.8451) -> (37.7542, 29.404)
  line L129 (37.7542, 29.404) -> (36.129, 29.404)
  spline S224 degree 2 poles (36.129, 29.404) (36.1487, 29.2558) (36.1636, 28.9693) (36.1636, 28.8507) knots 0 0 0 1 2 2 2
  spline S225 degree 2 poles (36.1636, 28.8507) (36.1636, 28.3814) (36.0104, 27.7343) (35.7832, 27.4379) knots 0 0 0 1 2 2 2
  spline S226 degree 2 poles (35.7832, 27.4379) (35.5559, 27.1365) (34.8643, 26.8105) (34.311, 26.8105) knots 0 0 0 1 2 2 2
  spline S227 degree 2 poles (35.4225, 22.1372) (33.7825, 22.1372) (32.2461, 23.0907) (32.2461, 24.0836) knots 0 0 0 1 2 2 2
  spline S228 degree 2 poles (32.2461, 24.0836) (32.2461, 25.0914) (33.8121, 26.0349) (35.4176, 26.0349) knots 0 0 0 1 2 2 2
  spline S229 degree 2 poles (35.4176, 26.0349) (37.0676, 26.0349) (38.594, 25.0815) (38.594, 24.0836) knots 0 0 0 1 2 2 2
  spline S230 degree 2 poles (38.594, 24.0836) (38.594, 23.0808) (37.0132, 22.1372) (35.4225, 22.1372) knots 0 0 0 1 2 2 2
  spline S231 degree 2 poles (33.5651, 23.1845) (33.8664, 23.066) (34.7952, 22.9672) (35.4225, 22.9672) knots 0 0 0 1 2 2 2
  spline S232 degree 2 poles (35.4225, 22.9672) (36.0499, 22.9672) (36.9737, 23.066) (37.2849, 23.1895) knots 0 0 0 1 2 2 2
  spline S233 degree 2 poles (37.2849, 23.1895) (37.5962, 23.313) (37.9173, 23.7427) (37.9173, 24.0836) knots 0 0 0 1 2 2 2
  spline S234 degree 2 poles (37.9173, 24.0836) (37.9173, 24.4245) (37.5962, 24.8641) (37.2751, 24.9926) knots 0 0 0 1 2 2 2
  spline S235 degree 2 poles (37.2751, 24.9926) (36.9638, 25.1161) (36.0154, 25.205) (35.4176, 25.205) knots 0 0 0 1 2 2 2
  spline S236 degree 2 poles (35.4176, 25.205) (34.7754, 25.205) (33.9158, 25.126) (33.5799, 24.9975) knots 0 0 0 1 2 2 2
  spline S237 degree 2 poles (33.5799, 24.9975) (33.2638, 24.879) (32.9229, 24.4393) (32.9229, 24.0836) knots 0 0 0 1 2 2 2
  spline S238 degree 2 poles (32.9229, 24.0836) (32.9229, 23.7477) (33.244, 23.308) (33.5651, 23.1845) knots 0 0 0 1 2 2 2
  spline S239 degree 2 poles (35.4225, 17.5628) (33.7825, 17.5628) (32.2461, 18.5162) (32.2461, 19.5091) knots 0 0 0 1 2 2 2
  spline S240 degree 2 poles (32.2461, 19.5091) (32.2461, 20.5169) (33.8121, 21.4604) (35.4176, 21.4604) knots 0 0 0 1 2 2 2
  spline S241 degree 2 poles (35.4176, 21.4604) (37.0676, 21.4604) (38.594, 20.507) (38.594, 19.5091) knots 0 0 0 1 2 2 2
  spline S242 degree 2 poles (38.594, 19.5091) (38.594, 18.5063) (37.0132, 17.5628) (35.4225, 17.5628) knots 0 0 0 1 2 2 2
  spline S243 degree 2 poles (33.5651, 18.61) (33.8664, 18.4915) (34.7952, 18.3927) (35.4225, 18.3927) knots 0 0 0 1 2 2 2
  spline S244 degree 2 poles (35.4225, 18.3927) (36.0499, 18.3927) (36.9737, 18.4915) (37.2849, 18.615) knots 0 0 0 1 2 2 2
  spline S245 degree 2 poles (37.2849, 18.615) (37.5962, 18.7385) (37.9173, 19.1683) (37.9173, 19.5091) knots 0 0 0 1 2 2 2
  spline S246 degree 2 poles (37.9173, 19.5091) (37.9173, 19.85) (37.5962, 20.2897) (37.2751, 20.4181) knots 0 0 0 1 2 2 2
  spline S247 degree 2 poles (37.2751, 20.4181) (36.9638, 20.5416) (36.0154, 20.6305) (35.4176, 20.6305) knots 0 0 0 1 2 2 2
  spline S248 degree 2 poles (35.4176, 20.6305) (34.7754, 20.6305) (33.9158, 20.5515) (33.5799, 20.423) knots 0 0 0 1 2 2 2
  spline S249 degree 2 poles (33.5799, 20.423) (33.2638, 20.3045) (32.9229, 19.8648) (32.9229, 19.5091) knots 0 0 0 1 2 2 2
  spline S250 degree 2 poles (32.9229, 19.5091) (32.9229, 19.1732) (33.244, 18.7336) (33.5651, 18.61) knots 0 0 0 1 2 2 2
  line L130 (32.3745, 13.3292) -> (32.3745, 16.3031)
  line L131 (32.3745, 16.3031) -> (32.997, 16.3031)
  line L132 (32.997, 16.3031) -> (32.997, 15.1965)
  line L133 (32.997, 15.1965) -> (37.0824, 15.1965)
  line L134 (37.0824, 15.1965) -> (37.0824, 16.3031)
  line L135 (37.0824, 16.3031) -> (37.6406, 16.3031)
  spline S251 degree 2 poles (37.6406, 16.3031) (37.6406, 15.6757) (37.9963, 15.0829) (38.4903, 15.0433) knots 0 0 0 1 2 2 2
  line L136 (38.4903, 15.0433) -> (38.4903, 14.411)
  line L137 (38.4903, 14.411) -> (32.997, 14.411)
  line L138 (32.997, 14.411) -> (32.997, 13.3292)
  line L139 (32.997, 13.3292) -> (32.3745, 13.3292)
  spline S252 degree 2 poles (24.2741, 72.3897) (23.8345, 72.3897) (23.0836, 72.6713) (22.8069, 72.9282) knots 0 0 0 1 2 2 2
  spline S253 degree 2 poles (22.8069, 72.9282) (22.5303, 73.1851) (22.2092, 73.9508) (22.2092, 74.425) knots 0 0 0 1 2 2 2
  spline S254 degree 2 poles (22.2092, 74.425) (22.2092, 74.8597) (22.4019, 75.7094) (22.555, 76.0206) knots 0 0 0 1 2 2 2
  line L140 (22.555, 76.0206) -> (23.4195, 76.0206)
  line L141 (23.4195, 76.0206) -> (23.4195, 75.9614)
  spline S255 degree 2 poles (23.4195, 75.9614) (23.3504, 75.8675) (23.1725, 75.5168) (23.0935, 75.3043) knots 0 0 0 1 2 2 2
  spline S256 degree 2 poles (23.0935, 75.3043) (23.0095, 75.0623) (22.9156, 74.6621) (22.9156, 74.4102) knots 0 0 0 1 2 2 2
  spline S257 degree 2 poles (22.9156, 74.4102) (22.9156, 74.1632) (23.0935, 73.6988) (23.2861, 73.5309) knots 0 0 0 1 2 2 2
  spline S258 degree 2 poles (23.2861, 73.5309) (23.4689, 73.3777) (23.953, 73.2196) (24.2791, 73.2196) knots 0 0 0 1 2 2 2
  spline S259 degree 2 poles (24.2791, 73.2196) (24.6051, 73.2196) (25.0201, 73.3975) (25.1584, 73.5654) knots 0 0 0 1 2 2 2
  spline S260 degree 2 poles (25.1584, 73.5654) (25.3115, 73.7383) (25.44, 74.2521) (25.44, 74.5633) knots 0 0 0 1 2 2 2
  spline S261 degree 2 poles (25.44, 74.5633) (25.44, 74.8993) (25.3362, 75.5662) (25.2918, 75.7687) knots 0 0 0 1 2 2 2
  line L142 (25.2918, 75.7687) -> (28.4336, 75.7687)
  line L143 (28.4336, 75.7687) -> (28.4336, 72.4243)
  line L144 (28.4336, 72.4243) -> (27.7173, 72.4243)
  line L145 (27.7173, 72.4243) -> (27.7173, 74.9832)
  line L146 (27.7173, 74.9832) -> (26.0921, 74.9832)
  spline S262 degree 2 poles (26.0921, 74.9832) (26.1118, 74.835) (26.1267, 74.5485) (26.1267, 74.4299) knots 0 0 0 1 2 2 2
  spline S263 degree 2 poles (26.1267, 74.4299) (26.1267, 73.9606) (25.9735, 73.3135) (25.7463, 73.0171) knots 0 0 0 1 2 2 2
  spline S264 degree 2 poles (25.7463, 73.0171) (25.519, 72.7158) (24.8274, 72.3897) (24.2741, 72.3897) knots 0 0 0 1 2 2 2
  spline S265 degree 2 poles (22.2487, 70.0136) (22.2487, 70.6409) (22.965, 71.3474) (23.7406, 71.3474) knots 0 0 0 1 2 2 2
  line L147 (23.7406, 71.3474) -> (26.2749, 71.3474)
  line L148 (26.2749, 71.3474) -> (26.2749, 71.8661)
  line L149 (26.2749, 71.8661) -> (26.9121, 71.8661)
  line L150 (26.9121, 71.8661) -> (26.9121, 71.3474)
  line L151 (26.9121, 71.3474) -> (28.2262, 71.3474)
  line L152 (28.2262, 71.3474) -> (28.2262, 70.5767)
  line L153 (28.2262, 70.5767) -> (26.9121, 70.5767)
  line L154 (26.9121, 70.5767) -> (26.9121, 69.1589)
  line L155 (26.9121, 69.1589) -> (26.2749, 69.1589)
  line L156 (26.2749, 69.1589) -> (26.2749, 70.5767)
  line L157 (26.2749, 70.5767) -> (24.0963, 70.5767)
  spline S266 degree 2 poles (24.0963, 70.5767) (23.7505, 70.5767) (23.3701, 70.552) (23.2071, 70.468) knots 0 0 0 1 2 2 2
  spline S267 degree 2 poles (23.2071, 70.468) (23.0638, 70.3989) (22.9206, 70.0877) (22.9206, 69.8209) knots 0 0 0 1 2 2 2
  spline S268 degree 2 poles (22.9206, 69.8209) (22.9206, 69.6332) (23.0342, 69.2824) (23.0688, 69.2034) knots 0 0 0 1 2 2 2
  line L158 (23.0688, 69.2034) -> (23.0688, 69.1589)
  line L159 (23.0688, 69.1589) -> (22.3772, 69.1589)
  spline S269 degree 2 poles (22.3772, 69.1589) (22.3179, 69.3763) (22.2487, 69.8209) (22.2487, 70.0136) knots 0 0 0 1 2 2 2
  line L160 (22.3376, 64.9994) -> (22.3376, 65.7701)
  line L161 (22.3376, 65.7701) -> (24.946, 65.7701)
  spline S270 degree 2 poles (24.946, 65.7701) (25.2621, 65.7701) (25.8055, 65.8294) (25.9686, 65.9183) knots 0 0 0 1 2 2 2
  spline S271 degree 2 poles (25.9686, 65.9183) (26.1415, 66.0121) (26.3094, 66.3481) (26.3094, 66.6346) knots 0 0 0 1 2 2 2
  spline S272 degree 2 poles (26.3094, 66.6346) (26.3094, 66.9211) (26.0031, 67.5287) (25.7561, 67.8202) knots 0 0 0 1 2 2 2
  line L162 (25.7561, 67.8202) -> (22.3376, 67.8202)
  line L163 (22.3376, 67.8202) -> (22.3376, 68.5908)
  line L164 (22.3376, 68.5908) -> (28.7053, 68.5908)
  line L165 (28.7053, 68.5908) -> (28.7053, 67.8202)
  line L166 (28.7053, 67.8202) -> (26.4033, 67.8202)
  spline S273 degree 2 poles (26.4033, 67.8202) (26.7145, 67.4744) (27.0406, 66.8075) (27.0406, 66.432) knots 0 0 0 1 2 2 2
  spline S274 degree 2 poles (27.0406, 66.432) (27.0406, 65.7602) (26.1514, 64.9994) (25.3066, 64.9994) knots 0 0 0 1 2 2 2
  line L167 (25.3066, 64.9994) -> (22.3376, 64.9994)
  spline S275 degree 2 poles (22.229, 59.5407) (22.229, 60.2027) (22.5056, 61.1314) (22.7032, 61.5414) knots 0 0 0 1 2 2 2
  line L168 (22.7032, 61.5414) -> (23.7209, 61.5414)
  line L169 (23.7209, 61.5414) -> (23.7209, 61.4821)
  spline S276 degree 2 poles (23.7209, 61.4821) (23.3454, 61.082) (22.9304, 60.0693) (22.9304, 59.6) knots 0 0 0 1 2 2 2
  spline S277 degree 2 poles (22.9304, 59.6) (22.9304, 58.9281) (23.4887, 58.2415) (23.9481, 58.2415) knots 0 0 0 1 2 2 2
  spline S278 degree 2 poles (23.9481, 58.2415) (24.3137, 58.2415) (24.7681, 58.6021) (24.8818, 58.9923) knots 0 0 0 1 2 2 2
  spline S279 degree 2 poles (24.8818, 58.9923) (24.9608, 59.2739) (25.0695, 59.7432) (25.1584, 60.094) knots 0 0 0 1 2 2 2
  spline S280 degree 2 poles (25.1584, 60.094) (25.2424, 60.4101) (25.4943, 60.9091) (25.6969, 61.1017) knots 0 0 0 1 2 2 2
  spline S281 degree 2 poles (25.6969, 61.1017) (25.8994, 61.2895) (26.4428, 61.4969) (26.7985, 61.4969) knots 0 0 0 1 2 2 2
  spline S282 degree 2 poles (26.7985, 61.4969) (27.5395, 61.4969) (28.5423, 60.341) (28.5423, 59.4468) knots 0 0 0 1 2 2 2
  spline S283 degree 2 poles (28.5423, 59.4468) (28.5423, 58.9331) (28.3398, 58.0241) (28.1471, 57.6338) knots 0 0 0 1 2 2 2
  line L170 (28.1471, 57.6338) -> (27.1789, 57.6338)
  line L171 (27.1789, 57.6338) -> (27.1789, 57.6931)
  spline S284 degree 2 poles (27.1789, 57.6931) (27.4456, 57.9846) (27.8408, 58.8935) (27.8408, 59.3925) knots 0 0 0 1 2 2 2
  spline S285 degree 2 poles (27.8408, 59.3925) (27.8408, 59.9557) (27.3123, 60.6522) (26.8825, 60.6522) knots 0 0 0 1 2 2 2
  spline S286 degree 2 poles (26.8825, 60.6522) (26.4972, 60.6522) (26.0377, 60.2422) (25.934, 59.8569) knots 0 0 0 1 2 2 2
  spline S287 degree 2 poles (25.934, 59.8569) (25.8648, 59.6) (25.687, 58.854) (25.6129, 58.607) knots 0 0 0 1 2 2 2
  spline S288 degree 2 poles (25.6129, 58.607) (25.4202, 57.9796) (24.6446, 57.3967) (24.0765, 57.3967) knots 0 0 0 1 2 2 2
  spline S289 degree 2 poles (24.0765, 57.3967) (23.7159, 57.3967) (23.0243, 57.6882) (22.7822, 57.95) knots 0 0 0 1 2 2 2
  spline S290 degree 2 poles (22.7822, 57.95) (22.5155, 58.2415) (22.229, 58.9825) (22.229, 59.5407) knots 0 0 0 1 2 2 2
  spline S291 degree 2 poles (22.2339, 54.6451) (22.2339, 55.7418) (23.464, 56.9472) (24.6002, 56.9472) knots 0 0 0 1 2 2 2
  spline S292 degree 2 poles (24.6002, 56.9472) (25.7166, 56.9472) (27.0406, 55.7764) (27.0406, 54.8328) knots 0 0 0 1 2 2 2
  spline S293 degree 2 poles (27.0406, 54.8328) (27.0406, 54.408) (26.7936, 53.751) (26.5317, 53.5089) knots 0 0 0 1 2 2 2
  spline S294 degree 2 poles (26.5317, 53.5089) (26.2699, 53.2619) (25.5141, 53.0001) (24.9657, 53.0001) knots 0 0 0 1 2 2 2
  line L172 (24.9657, 53.0001) -> (24.5458, 53.0001)
  line L173 (24.5458, 53.0001) -> (24.5458, 56.1666)
  spline S295 degree 2 poles (24.5458, 56.1666) (23.7505, 56.1666) (22.9057, 55.3664) (22.9057, 54.655) knots 0 0 0 1 2 2 2
  spline S296 degree 2 poles (22.9057, 54.655) (22.9057, 54.4031) (23.0194, 53.914) (23.1083, 53.7164) knots 0 0 0 1 2 2 2
  spline S297 degree 2 poles (23.1083, 53.7164) (23.2071, 53.5089) (23.38, 53.2224) (23.459, 53.1285) knots 0 0 0 1 2 2 2
  line L174 (23.459, 53.1285) -> (23.459, 53.0841)
  line L175 (23.459, 53.0841) -> (22.6192, 53.0841)